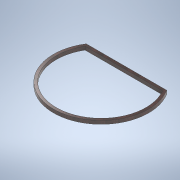
# Autodesk Inventor part: NestTop-ver2-1111-2021
Saved by Autodesk Inventor 2021 (Build 250183000, 183)
## iProperties
Created: 2021-03-02
Part Number: NestTop-ver2-1111-2021
Material: Generic
Document SubType Name: Modeling
Designer: CMurray
Density: 1 g/cm^3
Appearance: White Oak - Wild Berries
Author: CMurray
Autodesk Inventor part; units mm, degrees
ref_plane "YZ Plane" through (0, 0, 0) normal (1, 0, 0) x (0, 1, 0)
ref_plane "XZ Plane" through (0, 0, 0) normal (0, 1, 0) x (-1, 0, 0)
ref_plane "XY Plane" through (0, 0, 0) normal (0, 0, 1) x (1, 0, 0)
sketch "Sketch2" plane through (0, 0, 0) normal (0, 1, 0) x (-1, 0, 0)
  arc A0 (762, -479.9355) -> (-762, -479.9355) centre (0, 0) ccw
  line L0 (900.5455, 0) -> (762, 0)
  line L1 (762, -479.9355) -> (-762, -479.9355)
  dimension "d8" = 1524
  constraints: 4 end point, 3 point on circle, 1 centre point, 1 coincident, 1 horizontal
  measures "d8" distance of L1.start L1.end
extrude "Extrusion1" add sketch "Sketch2" along normal blind 63.5
sketch "Sketch9" plane through (0, 63.5, 0) normal (0, 1, 0) x (1, 0, 0)
  arc A0 (-762, 479.9355) -> (762, 479.9355) centre (0, 0) ccw
  line L0 (762, 479.9355) -> (-762, 479.9355) projected
  line L1 (-762, 479.9355) -> (762, 479.9355)
  arc A1 (-733.4235, 429.1355) -> (733.4235, 429.1355) centre (0, 0) ccw
  line L2 (-733.4235, 429.1355) -> (733.4235, 429.1355)
  dimension "d42" = 50.8
  constraints: 4 end point, 4 point on circle, 2 centre point, 1 coincident, 1 horizontal, 1 other
  measures "d42" radial gap between concentric circles of A0 A1
extrude "Extrusion10" cut sketch "Sketch9" against normal blind 76.2 contours L2 A1
body "Solid1"
